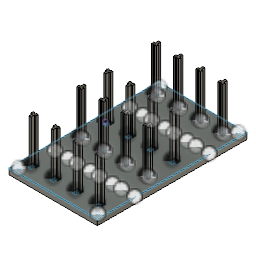
8 arduholder (Autodesk Fusion 360 design; units mm, degrees)
Autodesk Fusion 360 part; units mm, degrees
sketch "Sketch1" plane through (0, 0, 0) normal (0, 0, 1) x (1, 0, 0)
  line L0 (0, 0) -> (6, 0)
  line L1 (6, 0) -> (6, 3)
  line L2 (6, 3) -> (0, 3)
  line L3 (0, 3) -> (0, 0)
  line L4 (2.0299, 3) -> (3.8299, 3)
  line L5 (3.8299, 3) -> (3.8299, 2.2)
  line L6 (3.8299, 2.2) -> (2.0299, 2.2)
  line L7 (2.0299, 2.2) -> (2.0299, 3)
  line L8 (-0.0239, 29.2) -> (15.9515, 29.2) construction
  line L9 (0, 55.4) -> (0, 58.4)
  line L10 (6, 55.4) -> (0, 55.4)
  line L11 (2.0299, 56.2) -> (2.0299, 55.4)
  line L12 (2.0299, 55.4) -> (3.8299, 55.4)
  line L13 (0, 58.4) -> (6, 58.4)
  line L14 (6, 58.4) -> (6, 55.4)
  line L15 (3.8299, 56.2) -> (2.0299, 56.2)
  line L16 (3.8299, 55.4) -> (3.8299, 56.2)
  line L17 (1.8114, 0) -> (4.3712, 0)
  line L18 (4.3712, 0) -> (4.3712, -3.9406)
  line L19 (4.3712, -3.9406) -> (1.8114, -3.9406)
  line L20 (1.8114, -3.9406) -> (1.8114, 0)
  line L21 (1.8114, 62.3406) -> (1.8114, 58.4)
  line L22 (4.3712, 58.4) -> (4.3712, 62.3406)
  line L23 (4.3712, 62.3406) -> (1.8114, 62.3406)
  line L24 (31.0379, 0) -> (31.0379, -3.9406)
  line L25 (32.6667, 3) -> (26.6667, 3)
  line L26 (26.6667, 3) -> (26.6667, 0)
  line L27 (26.6667, 0) -> (32.6667, 0)
  line L28 (31.0379, -3.9406) -> (28.478, -3.9406)
  line L29 (28.6965, 55.4) -> (30.4965, 55.4)
  line L30 (28.6965, 3) -> (30.4965, 3)
  line L31 (31.0379, 62.3406) -> (28.478, 62.3406)
  line L32 (28.478, 62.3406) -> (28.478, 58.4)
  line L33 (28.478, -3.9406) -> (28.478, 0)
  line L34 (30.4965, 2.2) -> (28.6965, 2.2)
  line L35 (26.6667, 58.4) -> (32.6667, 58.4)
  line L36 (30.4965, 56.2) -> (28.6965, 56.2)
  line L37 (28.6965, 2.2) -> (28.6965, 3)
  line L38 (26.6667, 55.4) -> (26.6667, 58.4)
  line L39 (31.0379, 58.4) -> (31.0379, 62.3406)
  line L40 (32.6667, 55.4) -> (26.6667, 55.4)
  line L41 (26.6428, 29.2) -> (42.6181, 29.2) construction
  line L42 (30.4965, 55.4) -> (30.4965, 56.2)
  line L43 (30.4965, 3) -> (30.4965, 2.2)
  line L44 (32.6667, 0) -> (32.6667, 3)
  line L45 (28.478, 0) -> (31.0379, 0)
  line L46 (32.6667, 58.4) -> (32.6667, 55.4)
  line L47 (28.6965, 56.2) -> (28.6965, 55.4)
  line L48 (57.7046, 0) -> (57.7046, -3.9406)
  line L49 (59.3333, 3) -> (53.3333, 3)
  line L50 (53.3333, 3) -> (53.3333, 0)
  line L51 (53.3333, 0) -> (59.3333, 0)
  line L52 (57.7046, -3.9406) -> (55.1447, -3.9406)
  line L53 (55.3632, 55.4) -> (57.1632, 55.4)
  line L54 (55.3632, 3) -> (57.1632, 3)
  line L55 (57.7046, 62.3406) -> (55.1447, 62.3406)
  line L56 (55.1447, 62.3406) -> (55.1447, 58.4)
  line L57 (55.1447, -3.9406) -> (55.1447, 0)
  line L58 (57.1632, 2.2) -> (55.3632, 2.2)
  line L59 (53.3333, 58.4) -> (59.3333, 58.4)
  line L60 (57.1632, 56.2) -> (55.3632, 56.2)
  line L61 (55.3632, 2.2) -> (55.3632, 3)
  line L62 (53.3333, 55.4) -> (53.3333, 58.4)
  line L63 (57.7046, 58.4) -> (57.7046, 62.3406)
  line L64 (59.3333, 55.4) -> (53.3333, 55.4)
  line L65 (53.3095, 29.2) -> (69.2848, 29.2) construction
  line L66 (57.1632, 55.4) -> (57.1632, 56.2)
  line L67 (57.1632, 3) -> (57.1632, 2.2)
  line L68 (59.3333, 0) -> (59.3333, 3)
  line L69 (55.1447, 0) -> (57.7046, 0)
  line L70 (59.3333, 58.4) -> (59.3333, 55.4)
  line L71 (55.3632, 56.2) -> (55.3632, 55.4)
  line L72 (84.3712, 0) -> (84.3712, -3.9406)
  line L73 (86, 3) -> (80, 3)
  line L74 (80, 3) -> (80, 0)
  line L75 (80, 0) -> (86, 0)
  line L76 (84.3712, -3.9406) -> (81.8114, -3.9406)
  line L77 (82.0299, 55.4) -> (83.8299, 55.4)
  line L78 (82.0299, 3) -> (83.8299, 3)
  line L79 (84.3712, 62.3406) -> (81.8114, 62.3406)
  line L80 (81.8114, 62.3406) -> (81.8114, 58.4)
  line L81 (81.8114, -3.9406) -> (81.8114, 0)
  line L82 (83.8299, 2.2) -> (82.0299, 2.2)
  line L83 (80, 58.4) -> (86, 58.4)
  line L84 (83.8299, 56.2) -> (82.0299, 56.2)
  line L85 (82.0299, 2.2) -> (82.0299, 3)
  line L86 (80, 55.4) -> (80, 58.4)
  line L87 (84.3712, 58.4) -> (84.3712, 62.3406)
  line L88 (86, 55.4) -> (80, 55.4)
  line L89 (79.9761, 29.2) -> (95.9515, 29.2) construction
  line L90 (83.8299, 55.4) -> (83.8299, 56.2)
  line L91 (83.8299, 3) -> (83.8299, 2.2)
  line L92 (86, 0) -> (86, 3)
  line L93 (81.8114, 0) -> (84.3712, 0)
  line L94 (86, 58.4) -> (86, 55.4)
  line L95 (82.0299, 56.2) -> (82.0299, 55.4)
  line L96 (4.3712, -90) -> (4.3712, -93.9406)
  line L97 (6, -87) -> (0, -87)
  line L98 (0, -87) -> (0, -90)
  line L99 (0, -90) -> (6, -90)
  line L100 (4.3712, -93.9406) -> (1.8114, -93.9406)
  line L101 (2.0299, -34.6) -> (3.8299, -34.6)
  line L102 (2.0299, -87) -> (3.8299, -87)
  line L103 (4.3712, -27.6594) -> (1.8114, -27.6594)
  line L104 (1.8114, -27.6594) -> (1.8114, -31.6)
  line L105 (1.8114, -93.9406) -> (1.8114, -90)
  line L106 (3.8299, -87.8) -> (2.0299, -87.8)
  line L107 (0, -31.6) -> (6, -31.6)
  line L108 (3.8299, -33.8) -> (2.0299, -33.8)
  line L109 (2.0299, -87.8) -> (2.0299, -87)
  line L110 (0, -34.6) -> (0, -31.6)
  line L111 (4.3712, -31.6) -> (4.3712, -27.6594)
  line L112 (6, -34.6) -> (0, -34.6)
  line L113 (-0.0239, -60.8) -> (15.9515, -60.8) construction
  line L114 (3.8299, -34.6) -> (3.8299, -33.8)
  line L115 (3.8299, -87) -> (3.8299, -87.8)
  line L116 (6, -90) -> (6, -87)
  line L117 (1.8114, -90) -> (4.3712, -90)
  line L118 (6, -31.6) -> (6, -34.6)
  line L119 (2.0299, -33.8) -> (2.0299, -34.6)
  line L120 (31.0379, -90) -> (31.0379, -93.9406)
  line L121 (32.6667, -87) -> (26.6667, -87)
  line L122 (26.6667, -87) -> (26.6667, -90)
  line L123 (26.6667, -90) -> (32.6667, -90)
  line L124 (31.0379, -93.9406) -> (28.478, -93.9406)
  line L125 (28.6965, -34.6) -> (30.4965, -34.6)
  line L126 (28.6965, -87) -> (30.4965, -87)
  line L127 (31.0379, -27.6594) -> (28.478, -27.6594)
  line L128 (28.478, -27.6594) -> (28.478, -31.6)
  line L129 (28.478, -93.9406) -> (28.478, -90)
  line L130 (30.4965, -87.8) -> (28.6965, -87.8)
  line L131 (26.6667, -31.6) -> (32.6667, -31.6)
  line L132 (30.4965, -33.8) -> (28.6965, -33.8)
  line L133 (28.6965, -87.8) -> (28.6965, -87)
  line L134 (26.6667, -34.6) -> (26.6667, -31.6)
  line L135 (31.0379, -31.6) -> (31.0379, -27.6594)
  line L136 (32.6667, -34.6) -> (26.6667, -34.6)
  line L137 (26.6428, -60.8) -> (42.6181, -60.8) construction
  line L138 (30.4965, -34.6) -> (30.4965, -33.8)
  line L139 (30.4965, -87) -> (30.4965, -87.8)
  line L140 (32.6667, -90) -> (32.6667, -87)
  line L141 (28.478, -90) -> (31.0379, -90)
  line L142 (32.6667, -31.6) -> (32.6667, -34.6)
  line L143 (28.6965, -33.8) -> (28.6965, -34.6)
  line L144 (57.7046, -90) -> (57.7046, -93.9406)
  line L145 (59.3333, -87) -> (53.3333, -87)
  line L146 (53.3333, -87) -> (53.3333, -90)
  line L147 (53.3333, -90) -> (59.3333, -90)
  line L148 (57.7046, -93.9406) -> (55.1447, -93.9406)
  line L149 (55.3632, -34.6) -> (57.1632, -34.6)
  line L150 (55.3632, -87) -> (57.1632, -87)
  line L151 (57.7046, -27.6594) -> (55.1447, -27.6594)
  line L152 (55.1447, -27.6594) -> (55.1447, -31.6)
  line L153 (55.1447, -93.9406) -> (55.1447, -90)
  line L154 (57.1632, -87.8) -> (55.3632, -87.8)
  line L155 (53.3333, -31.6) -> (59.3333, -31.6)
  line L156 (57.1632, -33.8) -> (55.3632, -33.8)
  line L157 (55.3632, -87.8) -> (55.3632, -87)
  line L158 (53.3333, -34.6) -> (53.3333, -31.6)
  line L159 (57.7046, -31.6) -> (57.7046, -27.6594)
  line L160 (59.3333, -34.6) -> (53.3333, -34.6)
  line L161 (53.3095, -60.8) -> (69.2848, -60.8) construction
  line L162 (57.1632, -34.6) -> (57.1632, -33.8)
  line L163 (57.1632, -87) -> (57.1632, -87.8)
  line L164 (59.3333, -90) -> (59.3333, -87)
  line L165 (55.1447, -90) -> (57.7046, -90)
  line L166 (59.3333, -31.6) -> (59.3333, -34.6)
  line L167 (55.3632, -33.8) -> (55.3632, -34.6)
  line L168 (84.3712, -90) -> (84.3712, -93.9406)
  line L169 (86, -87) -> (80, -87)
  line L170 (80, -87) -> (80, -90)
  line L171 (80, -90) -> (86, -90)
  line L172 (84.3712, -93.9406) -> (81.8114, -93.9406)
  line L173 (82.0299, -34.6) -> (83.8299, -34.6)
  line L174 (82.0299, -87) -> (83.8299, -87)
  line L175 (84.3712, -27.6594) -> (81.8114, -27.6594)
  line L176 (81.8114, -27.6594) -> (81.8114, -31.6)
  line L177 (81.8114, -93.9406) -> (81.8114, -90)
  line L178 (83.8299, -87.8) -> (82.0299, -87.8)
  line L179 (80, -31.6) -> (86, -31.6)
  line L180 (83.8299, -33.8) -> (82.0299, -33.8)
  line L181 (82.0299, -87.8) -> (82.0299, -87)
  line L182 (80, -34.6) -> (80, -31.6)
  line L183 (84.3712, -31.6) -> (84.3712, -27.6594)
  line L184 (86, -34.6) -> (80, -34.6)
  line L185 (79.9761, -60.8) -> (95.9515, -60.8) construction
  line L186 (83.8299, -34.6) -> (83.8299, -33.8)
  line L187 (83.8299, -87) -> (83.8299, -87.8)
  line L188 (86, -90) -> (86, -87)
  line L189 (81.8114, -90) -> (84.3712, -90)
  line L190 (86, -31.6) -> (86, -34.6)
  line L191 (82.0299, -33.8) -> (82.0299, -34.6)
  line L192 (-9.4526, 73.5706) -> (96.9618, 73.5706)
  line L193 (96.9618, 73.5706) -> (96.9618, -106.6917)
  line L194 (96.9618, -106.6917) -> (-9.4526, -106.6917)
  line L195 (-9.4526, -106.6917) -> (-9.4526, 73.5706)
  circle A0 centre (91.4576, 68.5251) radius 2
  circle A1 centre (-3.5424, 68.5251) radius 2
  circle A2 centre (91.4576, -100.4749) radius 2
  circle A3 centre (-3.5424, -100.4749) radius 2
  point P0 (0, 58.4)
  point P1 (26.6667, 0)
  point P2 (26.6667, 58.4)
  point P3 (53.3333, 0)
  point P4 (53.3333, 58.4)
  point P5 (80, 0)
  point P6 (80, 58.4)
  point P7 (0, -90)
  point P8 (0, -31.6)
  point P9 (26.6667, -90)
  point P10 (26.6667, -31.6)
  point P11 (53.3333, -90)
  point P12 (53.3333, -31.6)
  point P13 (80, -90)
  point P14 (80, -31.6)
  dimension "d1" = 6
  dimension "d2" = 3
  dimension "d3" = 1.8
  dimension "d4" = 0.8
  dimension "d10" = 2.0299
  dimension "d11" = 2.1701
  dimension "d12" = 27
  dimension "d15" = 80
  dimension "d16" = -90
  dimension "d17" = 180.2623
  dimension "d18" = 106.4144
  dimension "d19" = 4
  dimension "d22" = -95
  dimension "d23" = -169
  constraint horizontal L0
  constraint vertical L1
  constraint horizontal L2
  constraint vertical L3
  constraint coincident L0.start L3.end
  constraint horizontal L4
  constraint vertical L5
  constraint horizontal L6
  constraint vertical L7
  constraint coincident L2 L4.start
  constraint horizontal L8
  constraint symmetric L0.start L8 L9.end
  constraint symmetric L0.start L8 P0
  constraint symmetric L0.end L8 L13.end
  constraint symmetric L1.end L8 L10.start
  constraint symmetric L2.end L8 L9.start
  constraint symmetric L4.start L8 L11.end
  constraint symmetric L4.end L8 L12.end
  constraint symmetric L5.end L8 L15.start
  constraint symmetric L6.end L8 L11.start
  constraint horizontal L17
  constraint vertical L18
  constraint horizontal L19
  constraint vertical L20
  constraint coincident L0 L17.start
  constraint symmetric L8 L17.start L21.end
  constraint symmetric L8 L17.end L22.start
  constraint symmetric L8 L18.end L22.end
  constraint symmetric L8 L19.end L21.start
  constraint horizontal L192
  constraint vertical L193
  constraint horizontal L194
  constraint vertical L195
  measures "d1" distance of L0.start L0.end
  measures "d2" distance of L0.start L2.end
  measures "d3" distance of L4.start L4.end
  measures "d4" distance of L4.start L6.end
  measures "d10" distance of L3 L7
  measures "d11" distance of L1 L5
  measures "d12" distance of L6.end L8
  measures "d17" distance of L192 L194
  measures "d18" distance of L193 L195
  measures "d19" diameter of A0
extrude "Extrude1" add sketch "Sketch1" along normal blind 54 contours L0 L1 L2 L3 L5 L6 L7 L17 | L0 L17 L18 L19 L20 | L9 L10 L11 L13 L14 L15 L16 | L13 L21 L22 L23 | L24 L27 L28 L33 L45 | L25 L26 L27 L34 L37 L43 L44 L45 | L35 L36 L38 L40 L42 L46 L47 | L31 L32 L35 L39 | L48 L51 L52 L57 L69 | L49 L50 L51 L58 L61 L67 L68 L69 | L59 L60 L62 L64 L66 L70 L71 | L55 L56 L59 L63 | L72 L75 L76 L81 L93 | L73 L74 L75 L82 L85 L91 L92 L93 | L83 L84 L86 L88 L90 L94 L95 | L79 L80 L83 L87 | L96 L99 L100 L105 L117 | L97 L98 L99 L106 L109 L115 L116 L117 | L107 L108 L110 L112 L114 L118 L119 | L103 L104 L107 L111 | L120 L123 L124 L129 L141 | L121 L122 L123 L130 L133 L139 L140 L141 | L131 L132 L134 L136 L138 L142 L143 | L127 L128 L131 L135 | L144 L147 L148 L153 L165 | L145 L146 L147 L154 L157 L163 L164 L165 | L155 L156 L158 L160 L162 L166 L167 | L151 L152 L155 L159 | L168 L171 L172 L177 L189 | L169 L170 L171 L178 L181 L187 L188 L189 | L179 L180 L182 L184 L186 L190 L191 | L175 L176 L179 L183 makes body 1 at (55.1447, 61.0271, 18) makes body 2 at (31.0379, -1.3135, 18) makes body 3 at (55.1447, -28.9729, 18) makes body 4 at (4.3712, -91.3135, 18) makes body 5 at (31.0379, -91.3135, 18) makes body 6 at (28.478, -28.9729, 18) makes body 7 at (55.1447, -2.6271, 18) makes body 8 at (28.478, 61.0271, 18) makes body 9 at (81.8114, 61.0271, 18) makes body 10 at (1.8114, -2.6271, 18) makes body 11 at (81.8114, -28.9729, 18) makes body 12 at (57.7046, -91.3135, 18) makes body 13 at (81.8114, -92.6271, 18) makes body 14 at (1.8114, -28.9729, 18) makes body 15 at (84.3712, -1.3135, 18) makes body 16 at (1.8114, 61.0271, 18)
extrude "Extrude2" add sketch "Sketch1" against normal blind 7 contours L0 L1 L2 L3 L5 L6 L7 L17 | L0 L17 L18 L19 L20 | L2 L4 L5 L6 L7 | L9 L10 L11 L13 L14 L15 L16 | L10 L11 L12 L15 L16 | L13 L21 L22 L23 | L24 L27 L28 L33 L45 | L25 L26 L27 L34 L37 L43 L44 L45 | L25 L30 L34 L37 L43 | L29 L36 L40 L42 L47 | L35 L36 L38 L40 L42 L46 L47 | L31 L32 L35 L39 | L48 L51 L52 L57 L69 | L49 L50 L51 L58 L61 L67 L68 L69 | L49 L54 L58 L61 L67 | L53 L60 L64 L66 L71 | L59 L60 L62 L64 L66 L70 L71 | L55 L56 L59 L63 | L72 L75 L76 L81 L93 | L73 L74 L75 L82 L85 L91 L92 L93 | L73 L78 L82 L85 L91 | L77 L84 L88 L90 L95 | L83 L84 L86 L88 L90 L94 L95 | L79 L80 L83 L87 | L96 L99 L100 L105 L117 | L97 L98 L99 L106 L109 L115 L116 L117 | L97 L102 L106 L109 L115 | L101 L108 L112 L114 L119 | L107 L108 L110 L112 L114 L118 L119 | L103 L104 L107 L111 | L120 L123 L124 L129 L141 | L121 L122 L123 L130 L133 L139 L140 L141 | L121 L126 L130 L133 L139 | L125 L132 L136 L138 L143 | L131 L132 L134 L136 L138 L142 L143 | L127 L128 L131 L135 | L144 L147 L148 L153 L165 | L145 L146 L147 L154 L157 L163 L164 L165 | L145 L150 L154 L157 L163 | L149 L156 L160 L162 L167 | L155 L156 L158 L160 L162 L166 L167 | L151 L152 L155 L159 | L168 L171 L172 L177 L189 | L169 L170 L171 L178 L181 L187 L188 L189 | L169 L174 L178 L181 L187 | L173 L180 L184 L186 L191 | L179 L180 L182 L184 L186 L190 L191 | L175 L176 L179 L183 | L192 L193 L194 L195 bodies 1 2 3 4 5 6 7 8 9 10 11 12 13 14 15 16
equation "d12 = ( 54 / 2 ) * 1 mm"
named bodies: "8arduholder"
